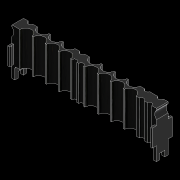
# Autodesk Inventor part: 3d_LM - Pinza 3
Saved by Autodesk Inventor 2018.3 (Build 223284000, 284)
## iProperties
Created: 2026-02-10
Part Number: 3d_LM - Pinza 3
Material: PA12 SLS 3D Print
Document SubType Name: Modeling
Designer: aca6
Density: 0.95 g/cm^3
Appearance: Black
Manufacturer-1: {"Name": "MATERIALISE NV", "PartNumber": "3d_LM - Pinza 3", "Link": ""}
Manufacturer-2: {"Name": "BERNARDO HENAREJOS ORENES (TECNOBRO)", "PartNumber": "3d_LM - Pinza 3", "Link": ""}
Manufacturer-3: {"Name": "", "PartNumber": "", "Link": ""}
Manufacturer-4: {"Name": "", "PartNumber": "", "Link": ""}
Manufacturer-5: {"Name": "", "PartNumber": "", "Link": ""}
Provider-1: {"Name": "", "PartNumber": "", "Link": ""}
Provider-2: {"Name": "", "PartNumber": "", "Link": ""}
Provider-3: {"Name": "", "PartNumber": "", "Link": ""}
Provider-4: {"Name": "", "PartNumber": "", "Link": ""}
Provider-5: {"Name": "", "PartNumber": "", "Link": ""}
Author: aca6
Comments: DIN-ISO-2768-mK
Autodesk Inventor part; units mm, degrees
ref_plane "YZ Plane" through (0, 0, 0) normal (1, 0, 0) x (0, 1, 0)
ref_plane "XZ Plane" through (0, 0, 0) normal (0, 1, 0) x (-1, 0, 0)
ref_plane "XY Plane" through (0, 0, 0) normal (0, 0, 1) x (1, 0, 0)
sketch "Sketch1" plane through (0, 0, 0) normal (0, 0, 1) x (1, 0, 0)
  line L0 (-25, 2) -> (-25, -2)
  line L1 (0, 0.3189) -> (0, -1.0844) construction
  line L2 (-25, 2) -> (25, 2)
  line L3 (25, 2) -> (25, -2)
  line L4 (25, -2) -> (-25, -2)
  line L5 (-1.8046, 0) -> (4.5195, 0) construction
  arc A0 (-23.4, 2) -> (-21.6, 2) centre (-22.5, 2) ccw
  arc A1 (-20.025, 2) -> (-15.975, 2) centre (-18, 2) ccw
  arc A2 (-15.525, 2) -> (-11.475, 2) centre (-13.5, 2) ccw
  arc A3 (-11.025, 2) -> (-6.975, 2) centre (-9, 2) ccw
  arc A4 (-5.4, 2) -> (-3.6, 2) centre (-4.5, 2) ccw
  arc A5 (-2.025, 2) -> (2.025, 2) centre (0, 2) ccw
  arc A6 (2.475, 2) -> (6.525, 2) centre (4.5, 2) ccw
  arc A7 (6.975, 2) -> (11.025, 2) centre (9, 2) ccw
  arc A8 (11.475, 2) -> (15.525, 2) centre (13.5, 2) ccw
  arc A9 (17.125, 2) -> (18.875, 2) centre (18, 2) ccw
  arc A10 (21.625, 2) -> (23.375, 2) centre (22.5, 2) ccw
  arc A11 (-18.225, -2) -> (-22.275, -2) centre (-20.25, -2) ccw
  arc A12 (-13.725, -2) -> (-17.775, -2) centre (-15.75, -2) ccw
  arc A13 (-9.225, -2) -> (-13.275, -2) centre (-11.25, -2) ccw
  arc A14 (-4.725, -2) -> (-8.775, -2) centre (-6.75, -2) ccw
  arc A15 (-2.535, -2) -> (-4.255, -2) centre (-3.395, -2) ccw
  arc A16 (-0.245, -2) -> (-1.965, -2) centre (-1.105, -2) ccw
  arc A17 (4.275, -2) -> (0.225, -2) centre (2.25, -2) ccw
  arc A18 (8.775, -2) -> (4.725, -2) centre (6.75, -2) ccw
  arc A19 (13.275, -2) -> (9.225, -2) centre (11.25, -2) ccw
  arc A20 (17.775, -2) -> (13.725, -2) centre (15.75, -2) ccw
  arc A21 (20.675, -2) -> (18.925, -2) centre (19.8, -2) ccw
  arc A22 (23.375, -2) -> (21.625, -2) centre (22.5, -2) ccw
  point P0 (0, 0)
  dimension "d0" = 4
  dimension "d1" = 50
  dimension "d2" = 2.5
  dimension "d3" = 4.5
  dimension "d4" = 4.5
  dimension "d5" = 4.5
  dimension "d6" = 4.5
  dimension "d7" = 4.5
  dimension "d8" = 4.5
  dimension "d10" = 4.5
  dimension "d11" = 4.5
  dimension "d12" = 4.5
  dimension "d13" = 4.5
  dimension "d14" = 1.8
  dimension "d15" = 4.05
  dimension "d16" = 4.05
  dimension "d17" = 4.05
  dimension "d18" = 1.8
  dimension "d19" = 4.05
  dimension "d20" = 4.05
  dimension "d21" = 4.05
  dimension "d22" = 4.05
  dimension "d23" = 1.75
  dimension "d24" = 1.75
  dimension "d25" = 4.05
  dimension "d27" = 4.5
  dimension "d28" = 4.5
  dimension "d29" = 4.5
  dimension "d30" = 3.355
  dimension "d31" = 2.29
  dimension "d32" = 3.355
  dimension "d33" = 4.5
  dimension "d34" = 4.5
  dimension "d35" = 4.5
  dimension "d37" = 1.75
  dimension "d38" = 4.05
  dimension "d39" = 4.05
  dimension "d40" = 4.05
  dimension "d41" = 4.05
  dimension "d42" = 1.72
  dimension "d43" = 1.72
  dimension "d44" = 4.05
  dimension "d45" = 4.05
  dimension "d46" = 4.05
  dimension "d47" = 1.75
  dimension "d48" = 2.7
  dimension "d136" = 2.5
  dimension "d143" = 4.05
  constraints: 46 point on circle, 23 centre point, 8 end point, 5 vertical, 3 horizontal, 78 other
  measures "d0" distance of L0.start L0.end
  measures "d1" distance of L0.start L3.start
  measures "d2" distance from line of L0 A0.centre
  measures "d3" distance of A1.centre A0.centre
  measures "d4" distance of A1.centre A2.centre
  measures "d5" distance of A3.centre A2.centre
  measures "d6" distance of A4.centre A3.centre
  measures "d7" distance of A5.centre A4.centre
  measures "d8" distance of A6.centre A5.centre
  measures "d10" distance of A7.centre A6.centre
  measures "d11" distance of A8.centre A7.centre
  measures "d12" distance of A9.centre A8.centre
  measures "d13" distance of A10.centre A9.centre
  measures "d14" diameter of A0
  measures "d15" diameter of A1
  measures "d16" diameter of A2
  measures "d17" diameter of A3
  measures "d18" diameter of A4
  measures "d19" diameter of A5
  measures "d20" diameter of A6
  measures "d21" diameter of A7
  measures "d22" diameter of A8
  measures "d23" diameter of A9
  measures "d24" diameter of A10
  measures "d25" diameter of A11
  measures "d27" distance of A12.centre A11.centre
  measures "d28" distance of A13.centre A12.centre
  measures "d29" distance of A13.centre A14.centre
  measures "d30" distance of A15.centre A14.centre
  measures "d31" distance of A15.centre A16.centre
  measures "d32" distance of A17.centre A16.centre
  measures "d33" distance of A18.centre A17.centre
  measures "d34" distance of A19.centre A18.centre
  measures "d35" distance of A19.centre A20.centre
  measures "d37" diameter of A21
  measures "d38" diameter of A20
  measures "d39" diameter of A19
  measures "d40" diameter of A18
  measures "d41" diameter of A17
  measures "d42" diameter of A16
  measures "d43" diameter of A15
  measures "d44" diameter of A14
  measures "d45" diameter of A13
  measures "d46" diameter of A12
  measures "d47" diameter of A22
  measures "d48" distance of A22.centre A21.centre
  measures "d136" distance from line of L3 A22.centre
  measures "d143" distance of A20.centre A21.centre
extrude "Extrusion1" add sketch "Sketch1" along normal blind 12 contours L2 A0 A1 A2 A3 A4 A5 A6 A7 A8 A9 A10 L3 L4 A22 A21 A20 A19 A18 A17 A16 A15 A14 A13 A12 A11 L0
sketch "Sketch2" plane through (23.375, 2, 0) normal (0, 1, 0) x (1, 0, 0)
  circle A0 centre (3.025, -9.9997) radius 2
  line L0 (1.625, 0) -> (1.625, -12) projected
  line L1 (1.625, -12) -> (1.625, -11.428)
  point P0 (-23.375, 0)
  dimension "d51" = 4
  dimension "d52" = 0.572
  dimension "d55" = 1.4
  constraints: 2 end point, 1 point on line, 3 other
  measures "d52" distance of L0.end L1.end
  measures "d55" horizontal distance of L1.end point (3.025, -10)
extrude "Extrusion2" cut sketch "Sketch2" against normal blind 12.5
sketch "Sketch3" plane through (-25, 2, 0) normal (0, 1, 0) x (1, 0, 0)
  circle A0 centre (-1.4, -9.9997) radius 2
  line L0 (0, 0) -> (0, -12) projected
  line L1 (0, -12) -> (0, -11.428)
  point P0 (25, 0)
  dimension "d58" = 4
  dimension "d59" = 0.572
  dimension "d60" = 1.4
  constraints: 2 end point, 1 point on line, 3 other
  measures "d59" distance of L0.end L1.end
  measures "d60" horizontal distance of L1.end point (-1.4, -10)
extrude "Extrusion3" cut sketch "Sketch3" against normal blind 12.5
sketch "Sketch4" plane through (0, 0, 12) normal (0, 0, 1) x (1, 0, 0)
  line L0 (-22.4782, 2) -> (21.8218, 2)
  line L1 (21.8218, 2) -> (21.8218, 1.825)
  line L2 (21.8218, 1.825) -> (-22.4782, 1.825)
  line L3 (-22.4782, 1.825) -> (-22.4782, 2)
  line L4 (-20.025, 2) -> (-21.6, 2) projected
  line L5 (-25, 2) -> (-25, -2) projected
  line L6 (13.275, -2) -> (13.725, -2) projected
  line L7 (-21.5, -2) -> (-8, -2)
  line L8 (-8, -2) -> (-8, -1.825)
  line L9 (-8, -1.825) -> (-21.5, -1.825)
  line L10 (-21.5, -1.825) -> (-21.5, -2)
  line L11 (0.89, -2) -> (21.8842, -2)
  line L12 (21.8842, -2) -> (21.8842, -1.825)
  line L13 (21.8842, -1.825) -> (0.89, -1.825)
  line L14 (0.89, -1.825) -> (0.89, -2)
  line L15 (-13.725, -2) -> (-13.275, -2) projected
  line L16 (25, -2) -> (25, 2) projected
  point P0 (0, 0)
  point P1 (-20.8125, 2)
  point P2 (13.5, -2)
  point P3 (-13.5, -2)
  dimension "d63" = 0.175
  dimension "d64" = 44.3
  dimension "d65" = 2.5218
  dimension "d69" = 0.175
  dimension "d70" = 0.175
  dimension "d71" = 3.5
  dimension "d72" = 17
  dimension "d73" = 3.1158
  dimension "d74" = 24.11
  constraints: 24 end point, 6 parallel, 3 horizontal, 3 midpoint, 3 perpendicular, 3 point on line
  measures "d63" distance of L0.end L1.end
  measures "d64" distance of L0.start L0.end
  measures "d65" distance between parallel lines of L5 L3
  measures "d69" distance of L8.end L7.end
  measures "d70" distance of L12.end L11.end
  measures "d71" distance between parallel lines of L5 L10
  measures "d72" distance between parallel lines of L5 L8
  measures "d73" distance between parallel lines of L16 L12
  measures "d74" distance between parallel lines of L16 L14
extrude "Extrusion4" cut sketch "Sketch4" against normal blind 12.5
ref_plane "Work Plane1" through (0, 0, 0.5) normal (0, 0, -1) x (-1, 0, 0)
sketch "Sketch5" plane through (0, 0, 0.5) normal (0, 0, -1) x (-1, 0, 0)
  line L0 (25, 2) -> (25, -2) projected
  line L1 (25, 2) -> (25, 3.5)
  line L2 (25, 3.5) -> (24.5, 3.5)
  line L3 (24.5, 3.5) -> (24.1998, 2.7996)
  line L4 (24.1998, 2.7996) -> (24.3998, 2.7996)
  line L5 (24.3998, 2.7996) -> (24.3998, 2)
  line L6 (23.4, 2) -> (25, 2) projected
  line L7 (25, -2) -> (22.275, -2) projected
  line L8 (25, -2) -> (25, -3.5)
  line L9 (25, -3.5) -> (24.5, -3.5)
  line L10 (24.5, -3.5) -> (24.1998, -2.7996)
  line L11 (24.1998, -2.7996) -> (24.3998, -2.7996)
  line L12 (24.3998, -2.7996) -> (24.3998, -2)
  line L13 (0, 0) -> (0, 7.5844) construction
  line L14 (25, 2) -> (24.3998, 2)
  line L15 (25, -2) -> (24.3998, -2)
  line L16 (-25, 2) -> (-25, -2)
  line L17 (-25, 2) -> (-25, 3.5)
  line L18 (-25, 3.5) -> (-24.5, 3.5)
  line L19 (-24.5, 3.5) -> (-24.1998, 2.7996)
  line L20 (-24.1998, 2.7996) -> (-24.3998, 2.7996)
  line L21 (-24.3998, 2.7996) -> (-24.3998, 2)
  line L22 (-23.4, 2) -> (-25, 2)
  line L23 (-25, -2) -> (-22.275, -2)
  line L24 (-25, -2) -> (-25, -3.5)
  line L25 (-25, -3.5) -> (-24.5, -3.5)
  line L26 (-24.5, -3.5) -> (-24.1998, -2.7996)
  line L27 (-24.1998, -2.7996) -> (-24.3998, -2.7996)
  line L28 (-24.3998, -2.7996) -> (-24.3998, -2)
  line L29 (-25, 2) -> (-24.3998, 2)
  line L30 (-25, -2) -> (-24.3998, -2)
  dimension "d78" = 1.5
  dimension "d79" = 0.5
  dimension "d80" = 0.762
  dimension "d81" = 0.2
  dimension "d83" = 113.2
  dimension "d84" = 0.7996
  dimension "d85" = 1.5
  dimension "d86" = 0.5
  dimension "d87" = 113.2
  dimension "d88" = 0.2
  dimension "d89" = 0.762
  constraints: 56 end point, 14 symmetric about line, 6 vertical, 4 point on line, 2 parallel, 2 perpendicular, 1 collinear, 1 horizontal, 1 other
  measures "d78" distance of L0.start L1.end
  measures "d79" distance of L1.end L2.end
  measures "d80" distance of L2.end L3.end
  measures "d81" distance of L3.end L4.end
  measures "d83" angle of L2 L3
  measures "d84" distance of L4.end L5.end
  measures "d85" distance of L0.end L8.end
  measures "d86" distance of L8.end L9.end
  measures "d87" angle of L9 L10
  measures "d88" distance of L10.end L11.end
  measures "d89" distance of L9.end L10.end
extrude "Extrusion5" add sketch "Sketch5" against normal blind 6 contours L6 L5 L4 L3 L2 L1 | L8 L9 L10 L11 L12 L7
ref_plane "Work Plane2" through (0, 0, 0.8) normal (0, 0, -1) x (-1, 0, 0)
sketch "Sketch8" plane through (0, 0, 0.8) normal (0, 0, -1) x (-1, 0, 0)
  line L0 (25, 2) -> (25, 3.5)
  line L1 (25, 3.5) -> (24.5, 3.5)
  line L2 (24.5, 3.5) -> (24.1998, 2.7996)
  line L3 (24.1998, 2.7996) -> (24.3998, 2.7996)
  line L4 (24.3998, 2.7996) -> (24.3998, 2)
  line L5 (24.25, 2) -> (25, 2)
  line L6 (25, 2) -> (24.3998, 2)
  arc A0 (-2.0174, 1.825) -> (2.0174, 1.825) centre (0, 2) ccw projected
  line L7 (0, 2) -> (0, 7.911) construction
  line L8 (-24.25, 2) -> (-25, 2)
  line L9 (-25, 2) -> (-24.3998, 2)
  line L10 (-24.1998, 2.7996) -> (-24.3998, 2.7996)
  line L11 (-24.3998, 2.7996) -> (-24.3998, 2)
  line L12 (-25, 2) -> (-25, 3.5)
  line L13 (-25, 3.5) -> (-24.5, 3.5)
  line L14 (-24.5, 3.5) -> (-24.1998, 2.7996)
  point P0 (0, 0)
  dimension "d112" = 1.5
  dimension "d113" = 0.5
  dimension "d114" = 0.762
  dimension "d115" = 0.2
  dimension "d116" = 113.2
  dimension "d117" = 0.7996
  constraints: 30 end point, 7 symmetric about line, 4 vertical, 2 point on line, 1 collinear, 1 horizontal, 1 parallel, 1 other
  measures "d112" distance of L5.end L0.end
  measures "d113" distance of L0.end L1.end
  measures "d114" distance of L1.end L3.start
  measures "d115" distance of L3.start L3.end
  measures "d116" angle of L1 L2
  measures "d117" distance of L3.end L6.end
extrude "Extrusion8" add sketch "Sketch8" against normal blind 6 contours L8 L12 L13 L14 L10 L11
mirror "Mirror1" about plane through (0, 0, 0) normal (0, 1, 0) of "Extrusion8"
ref_plane "Work Plane3" through (0, 0, 1.3) normal (0, 0, -1) x (-1, 0, 0)
sketch "Sketch11" plane through (0, 0, 0) normal (0, 0, -1) x (-1, 0, 0)
  line L0 (-25, 2) -> (-24.4, 2) projected
  line L1 (-23.375, -2) -> (-25, -2) projected
  line L2 (-25, 2) -> (-24, 2)
  line L3 (-24, 2) -> (-24, -2)
  line L4 (-24, -2) -> (-25, -2)
  line L5 (-25, -2) -> (-25, 2)
  line L6 (25, 2) -> (25, -2) projected
  line L7 (25, -2) -> (22.275, -2) projected
  line L8 (25, 2) -> (24, 2)
  line L9 (24, 2) -> (24, -2)
  line L10 (24, -2) -> (25, -2)
  line L11 (25, -2) -> (25, 2)
  point P0 (0, 0)
  dimension "d145" = 1
  dimension "d146" = 1
  constraints: 16 end point, 4 parallel, 2 horizontal, 2 perpendicular, 2 point on line
  measures "d145" distance of L3.end L4.end
  measures "d146" distance of L10.end L9.end
extrude "Extrusion11" add sketch "Sketch11" along normal blind 2.005
fillet "Fillet1" radius 0.5 2 edges at (24, 0, 0) (-24, 0, 0)
sketch "Sketch12" plane through (0, 0, -2.005) normal (0, 0, -1) x (-1, 0, 0)
  line L0 (-25, 2) -> (-25, -2) projected
  line L1 (-24, -2) -> (-24, 2) projected
  line L2 (-25, 0.9) -> (-24, 0.9)
  line L3 (-24, 0.9) -> (-24, -0.8147)
  line L4 (-24, -0.8147) -> (-25, -0.8147)
  line L5 (-25, -0.8147) -> (-25, 0.9)
  line L6 (-24, 2) -> (-25, 2) projected
  line L7 (-23.375, -2) -> (-25, -2) projected
  line L8 (-25, -2) -> (-24, -2)
  line L9 (-24, -2) -> (-24, -0.9)
  line L10 (-24, -0.9) -> (-25, -0.9)
  line L11 (-25, -0.9) -> (-25, -2)
  line L12 (25, -2) -> (25, 2) projected
  line L13 (25, 2) -> (24, 2)
  line L14 (24, 2) -> (24, 0.9)
  line L15 (24, 0.9) -> (25, 0.9)
  line L16 (25, 0.9) -> (25, 2)
  line L17 (25, -2) -> (25, -3.5) projected
  line L18 (25, -2) -> (24, -2)
  line L19 (24, -2) -> (24, -0.9)
  line L20 (24, -0.9) -> (25, -0.9)
  line L21 (25, -0.9) -> (25, -2)
  point P0 (0, 0)
  dimension "d150" = 1.1
  dimension "d151" = 1.1
  dimension "d152" = 1
  dimension "d153" = 1.1
  dimension "d154" = 1
  dimension "d155" = 1.1
  constraints: 32 end point, 8 parallel, 4 horizontal, 4 perpendicular, 3 point on line
  measures "d150" distance between parallel lines of L6 L2
  measures "d151" distance between parallel lines of L7 L10
  measures "d152" distance of L15.end L14.end
  measures "d153" distance of L14.end L13.end
  measures "d154" distance of L19.end L20.end
  measures "d155" distance of L18.end L19.end
extrude "Extrusion12" add sketch "Sketch12" along normal blind 2 contours L6 L1 L2 L0 | L4 L1 L10 L0 | L10 L1 L7 L0 | L18 L19 L20 L12 | L15 L14 L13 L12
sketch "Sketch13" plane through (25, -2, 8.5714) normal (1, 0, 0) x (0, 0, -1)
  line L0 (12.5764, 0) -> (12.5764, 1.1853) projected
  line L1 (12.5764, 1.1853) -> (10.5764, 1.1853)
  line L2 (12.5764, 1.2003) -> (12.5764, 1.1853)
  line L3 (119.9448, 1.2) -> (10.5764, 1.2) construction
  line L4 (10.5764, 1.2) -> (12.5764, 1.2)
  line L5 (12.5764, 1.2) -> (12.5764, 1.1)
  line L6 (12.5764, 1.1) -> (10.5764, 1.1)
  line L7 (10.5764, 1.1) -> (10.5764, 1.2)
  point P0 (8.5714, 2)
  dimension "d159" = 0.1
  constraints: 12 end point, 2 horizontal, 2 parallel, 1 perpendicular, 1 point on line
  measures "d159" distance of L4.end L5.end
extrude "Extrusion13" cut sketch "Sketch13" against normal blind 10
body "Solid1"
